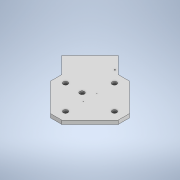
# Autodesk Inventor part: Base
Saved by Autodesk Inventor 2021 (Build 250183000, 183)
## iProperties
Created: 2021-06-02
Part Number: Base
Material: Genérico
Document SubType Name: Modeling
Designer: Marc
Density: 1 g/cm^3
Appearance: Valor por defecto
Author: Marc
Autodesk Inventor part; units mm, degrees
ref_plane "YZ Plane" through (0, 0, 0) normal (1, 0, 0) x (0, 1, 0)
ref_plane "XZ Plane" through (0, 0, 0) normal (0, 1, 0) x (-1, 0, 0)
ref_plane "XY Plane" through (0, 0, 0) normal (0, 0, 1) x (1, 0, 0)
sketch "Boceto1" plane through (0, 0, 0) normal (0, 1, 0) x (-1, 0, 0)
  line L0 (24.25, 145) -> (-24.25, 145)
  line L1 (-145, 24.25) -> (-145, -24.25)
  line L2 (-24.25, -145) -> (24.25, -145)
  line L3 (145, -24.25) -> (145, 24.25)
  line L4 (24.25, 145) -> (145, 24.25)
  line L5 (-24.25, -145) -> (-145, -24.25)
  line L6 (-145, 24.25) -> (-24.25, 145)
  line L7 (145, -24.25) -> (215.7107, -94.9607)
  line L8 (24.25, -145) -> (94.9607, -215.7107)
  line L9 (94.9607, -215.7107) -> (215.7107, -94.9607)
  point P0 (0, 0)
  constraints: 20 end point, 3 perpendicular, 2 parallel, 1 horizontal
extrude "Extrusión1" add sketch "Boceto1" against normal blind 16
sketch "Boceto2" plane through (0, 0, 0) normal (0, 1, 0) x (1, 0, 0)
  line L0 (-145, -24.25) -> (-145, 24.25) projected
  line L1 (24.25, -145) -> (-24.25, -145) projected
  line L2 (145, 24.25) -> (145, -24.25) projected
  line L3 (-24.25, 145) -> (24.25, 145) projected
  circle A0 centre (0, 105) radius 10
  circle A1 centre (-105, 0) radius 10
  circle A2 centre (105, 0) radius 10
  circle A3 centre (0, -105) radius 10
  circle A4 centre (0, 29) radius 1
  circle A5 centre (0, -29) radius 1
  circle A6 centre (-34, 0) radius 10
  circle A7 centre (-48.9987, 155.6066) radius 2.5
  dimension "d14" = 20
  dimension "d17" = 20
  dimension "d21" = 2
  dimension "d23" = 2
  dimension "d30" = 5
  constraints: 8 centre point
  measures "d14" diameter of A0
  measures "d17" diameter of A3
  measures "d21" diameter of A4
  measures "d23" diameter of A5
  measures "d30" diameter of A7
extrude "Extrusión2" cut sketch "Boceto2" against normal blind 20
thread "Rosca1" size "M5x0.8" class "6H" standard "ANSI Metric M Profile" full length
equation "\"d25\" = d14"
